Autodesk Fusion 360 part; units mm, degrees
note: some values were not read from the file. Set by a fixed rule: which sketch regions a step uses.
(part 10 of 59)
  spline S52 degree 5 poles (-23.3609, 32.8781) (-23.3596, 32.8757) (-23.3571, 32.871) (-23.3532, 32.8639) (-23.348, 32.8544) (-23.3416, 32.8426) (-23.3351, 32.8308) (-23.3287, 32.819) (-23.3222, 32.8073) (-23.3158, 32.7957) (-23.3094, 32.784) (-23.3029, 32.7724) (-23.2965, 32.7609) (-23.29, 32.7493) (-23.2836, 32.7379) (-23.2771, 32.7264) (-23.2707, 32.715) (-23.2643, 32.7036) (-23.2578, 32.6922) (-23.2514, 32.6809) (-23.245, 32.6697) (-23.2385, 32.6584) (-23.2321, 32.6472) (-23.2257, 32.636) (-23.2193, 32.6249) (-23.2128, 32.6138) (-23.2064, 32.6028) (-23.2, 32.5917) (-23.1936, 32.5808) (-23.1872, 32.5698) (-23.1807, 32.5589) (-23.1743, 32.548) (-23.1679, 32.5372) (-23.1615, 32.5264) (-23.1551, 32.5156) (-23.1487, 32.5049) (-23.1423, 32.4942) (-23.136, 32.4836) (-23.1296, 32.473) (-23.1232, 32.4624) (-23.1168, 32.4518) (-23.1104, 32.4413) (-23.1041, 32.4309) (-23.0977, 32.4205) (-23.0914, 32.4101) (-23.085, 32.3997) (-23.0786, 32.3894) (-23.0723, 32.3791) (-23.066, 32.3689) (-23.0596, 32.3587) (-23.0533, 32.3486) (-23.047, 32.3384) (-23.0406, 32.3284) (-23.0343, 32.3183) (-23.028, 32.3083) (-23.0217, 32.2984) (-23.0154, 32.2884) (-23.0091, 32.2785) (-23.0029, 32.2687) (-22.9966, 32.2589) (-22.9903, 32.2491) (-22.984, 32.2394) (-22.9778, 32.2297) (-22.9715, 32.22) (-22.9653, 32.2104) (-22.9591, 32.2009) (-22.9528, 32.1913) (-22.9466, 32.1818) (-22.9404, 32.1724) (-22.9342, 32.163) (-22.928, 32.1536) (-22.9218, 32.1443) (-22.9156, 32.135) (-22.9095, 32.1257) (-22.9033, 32.1165) (-22.8971, 32.1073) (-22.891, 32.0982) (-22.8849, 32.0891) (-22.8787, 32.0801) (-22.8726, 32.0711) (-22.8665, 32.0621) (-22.8604, 32.0532) (-22.8543, 32.0443) (-22.8483, 32.0354) (-22.8422, 32.0266) (-22.8361, 32.0179) (-22.8301, 32.0091) (-22.8241, 32.0005) (-22.818, 31.9918) (-22.812, 31.9832) (-22.806, 31.9747) (-22.8, 31.9662) (-22.7941, 31.9577) (-22.7881, 31.9493) (-22.7822, 31.9409) (-22.7762, 31.9325) (-22.7703, 31.9242) (-22.7644, 31.916) (-22.7585, 31.9078) (-22.7526, 31.8996) (-22.7467, 31.8914) (-22.7408, 31.8834) (-22.735, 31.8753) (-22.7292, 31.8673) (-22.7233, 31.8593) (-22.7175, 31.8514) (-22.7118, 31.8436) (-22.706, 31.8357) (-22.7002, 31.8279) (-22.6945, 31.8202) (-22.6887, 31.8125) (-22.683, 31.8048) (-22.6773, 31.7972) (-22.6716, 31.7897) (-22.666, 31.7821) (-22.6603, 31.7747) (-22.6547, 31.7672) (-22.6491, 31.7598) (-22.6435, 31.7525) (-22.6379, 31.7452) (-22.6323, 31.7379) (-22.6268, 31.7307) (-22.6212, 31.7236) (-22.6157, 31.7165) (-22.6102, 31.7094) (-22.6048, 31.7024) (-22.5993, 31.6954) (-22.5939, 31.6884) (-22.5884, 31.6815) (-22.583, 31.6747) (-22.5777, 31.6679) (-22.5723, 31.6611) (-22.567, 31.6544) (-22.5617, 31.6478) (-22.5564, 31.6412) (-22.5511, 31.6346) (-22.5458, 31.6281) (-22.5406, 31.6216) (-22.5354, 31.6152) (-22.5302, 31.6088) (-22.525, 31.6025) (-22.5199, 31.5962) (-22.5148, 31.59) (-22.5097, 31.5838) (-22.5046, 31.5776) (-22.4996, 31.5715) (-22.4945, 31.5655) (-22.4895, 31.5595) (-22.4846, 31.5536) (-22.4796, 31.5477) (-22.4747, 31.5418) (-22.4698, 31.536) (-22.4649, 31.5303) (-22.4601, 31.5246) (-22.4553, 31.5189) (-22.4505, 31.5133) (-22.4457, 31.5077) (-22.441, 31.5022) (-22.4363, 31.4968) (-22.4316, 31.4914) (-22.427, 31.486) (-22.4223, 31.4807) (-22.4177, 31.4755) (-22.4132, 31.4703) (-22.4087, 31.4651) (-22.4042, 31.46) (-22.3997, 31.455) (-22.3953, 31.45) (-22.3909, 31.4451) (-22.3865, 31.4402) (-22.3821, 31.4353) (-22.3778, 31.4306) (-22.3736, 31.4258) (-22.3693, 31.4211) (-22.3651, 31.4165) (-22.3609, 31.4119) (-22.3568, 31.4074) (-22.3527, 31.403) (-22.3486, 31.3986) (-22.3446, 31.3942) (-22.3406, 31.3899) (-22.3367, 31.3856) (-22.3328, 31.3814) (-22.3289, 31.3773) (-22.325, 31.3732) (-22.3212, 31.3692) (-22.3175, 31.3652) (-22.3138, 31.3613) (-22.3101, 31.3574) (-22.3065, 31.3536) (-22.3029, 31.3499) (-22.2993, 31.3462) (-22.2958, 31.3426) (-22.2923, 31.339) (-22.2889, 31.3355) (-22.2855, 31.332) (-22.2822, 31.3286) (-22.2789, 31.3252) (-22.2757, 31.322) (-22.2725, 31.3187) (-22.2693, 31.3156) (-22.2662, 31.3124) (-22.2632, 31.3094) (-22.2602, 31.3064) (-22.2572, 31.3035) (-22.2543, 31.3006) (-22.2515, 31.2978) (-22.2487, 31.2951) (-22.2459, 31.2924) (-22.2433, 31.2897) (-22.2406, 31.2872) (-22.238, 31.2847) (-22.2355, 31.2823) (-22.2331, 31.2799) (-22.2307, 31.2776) (-22.2283, 31.2753) (-22.226, 31.2732) (-22.2238, 31.271) (-22.2216, 31.269) (-22.2195, 31.267) (-22.2175, 31.2651) (-22.2155, 31.2632) (-22.2136, 31.2615) (-22.2117, 31.2597) (-22.2099, 31.2581) (-22.2082, 31.2565) (-22.2066, 31.255) (-22.205, 31.2536) (-22.2035, 31.2522) (-22.202, 31.2509) (-22.2007, 31.2497) (-22.1994, 31.2485) (-22.1982, 31.2474) (-22.197, 31.2464) (-22.196, 31.2455) (-22.195, 31.2446) (-22.1941, 31.2438) (-22.1933, 31.2431) (-22.1925, 31.2424) (-22.1919, 31.2419) (-22.1913, 31.2414) (-22.1909, 31.241) (-22.1907, 31.2408) (-22.1905, 31.2407) (-22.1904, 31.2406) knots -1 -1 -1 -1 -1 -1 -0.99583333 -0.99166667 -0.9875 -0.98333333 -0.97916667 -0.975 -0.97083333 -0.96666667 -0.9625 -0.95833333 -0.95416667 -0.95 -0.94583333 -0.94166667 -0.9375 -0.93333333 -0.92916667 -0.925 -0.92083333 -0.91666667 -0.9125 -0.90833333 -0.90416667 -0.9 -0.89583333 -0.89166667 -0.8875 -0.88333333 -0.87916667 -0.875 -0.87083333 -0.86666667 -0.8625 -0.85833333 -0.85416667 -0.85 -0.84583333 -0.84166667 -0.8375 -0.83333333 -0.82916667 -0.825 -0.82083333 -0.81666667 -0.8125 -0.80833333 -0.80416667 -0.8 -0.79583333 -0.79166667 -0.7875 -0.78333333 -0.77916667 -0.775 -0.77083333 -0.76666667 -0.7625 -0.75833333 -0.75416667 -0.75 -0.74583333 -0.74166667 -0.7375 -0.73333333 -0.72916667 -0.725 -0.72083333 -0.71666667 -0.7125 -0.70833333 -0.70416667 -0.7 -0.69583333 -0.69166667 -0.6875 -0.68333333 -0.67916667 -0.675 -0.67083333 -0.66666667 -0.6625 -0.65833333 -0.65416667 -0.65 -0.64583333 -0.64166667 -0.6375 -0.63333333 -0.62916667 -0.625 -0.62083333 -0.61666667 -0.6125 -0.60833333 -0.60416667 -0.6 -0.59583333 -0.59166667 -0.5875 -0.58333333 -0.57916667 -0.575 -0.57083333 -0.56666667 -0.5625 -0.55833333 -0.55416667 -0.55 -0.54583333 -0.54166667 -0.5375 -0.53333333 -0.52916667 -0.525 -0.52083333 -0.51666667 -0.5125 -0.50833333 -0.50416667 -0.5 -0.49583333 -0.49166667 -0.4875 -0.48333333 -0.47916667 -0.475 -0.47083333 -0.46666667 -0.4625 -0.45833333 -0.45416667 -0.45 -0.44583333 -0.44166667 -0.4375 -0.43333333 -0.42916667 -0.425 -0.42083333 -0.41666667 -0.4125 -0.40833333 -0.40416667 -0.4 -0.39583333 -0.39166667 -0.3875 -0.38333333 -0.37916667 -0.375 -0.37083333 -0.36666667 -0.3625 -0.35833333 -0.35416667 -0.35 -0.34583333 -0.34166667 -0.3375 -0.33333333 -0.32916667 -0.325 -0.32083333 -0.31666667 -0.3125 -0.30833333 -0.30416667 -0.3 -0.29583333 -0.29166667 -0.2875 -0.28333333 -0.27916667 -0.275 -0.27083333 -0.26666667 -0.2625 -0.25833333 -0.25416667 -0.25 -0.24583333 -0.24166667 -0.2375 -0.23333333 -0.22916667 -0.225 -0.22083333 -0.21666667 -0.2125 -0.20833333 -0.20416667 -0.2 -0.19583333 -0.19166667 -0.1875 -0.18333333 -0.17916667 -0.175 -0.17083333 -0.16666667 -0.1625 -0.15833333 -0.15416667 -0.15 -0.14583333 -0.14166667 -0.1375 -0.13333333 -0.12916667 -0.125 -0.12083333 -0.11666667 -0.1125 -0.10833333 -0.10416667 -0.1 -0.09583333 -0.09166667 -0.0875 -0.08333333 -0.07916667 -0.075 -0.07083333 -0.06666667 -0.0625 -0.05833333 -0.05416667 -0.05 -0.04583333 -0.04166667 -0.0375 -0.03333333 -0.02916667 -0.025 -0.02083333 -0.01666667 -0.0125 -0.00833333 -0.00416667 0 0 0 0 0 0
  line L120 (-10.8547, 39.1221) -> (-10.9659, 39.3948)
  spline S53 degree 5 poles (-10.0421, 41.8284) (-10.0422, 41.8257) (-10.0423, 41.8203) (-10.0425, 41.8122) (-10.0428, 41.8014) (-10.0431, 41.788) (-10.0434, 41.7745) (-10.0437, 41.7612) (-10.044, 41.7478) (-10.0442, 41.7345) (-10.0445, 41.7212) (-10.0447, 41.7079) (-10.0449, 41.6947) (-10.0451, 41.6815) (-10.0453, 41.6683) (-10.0454, 41.6551) (-10.0455, 41.642) (-10.0457, 41.629) (-10.0458, 41.6159) (-10.0458, 41.6029) (-10.0459, 41.5899) (-10.046, 41.577) (-10.046, 41.5641) (-10.046, 41.5512) (-10.046, 41.5383) (-10.046, 41.5255) (-10.046, 41.5127) (-10.0459, 41.5) (-10.0458, 41.4872) (-10.0458, 41.4745) (-10.0457, 41.4619) (-10.0456, 41.4493) (-10.0454, 41.4367) (-10.0453, 41.4241) (-10.0451, 41.4116) (-10.0449, 41.3991) (-10.0448, 41.3867) (-10.0445, 41.3743) (-10.0443, 41.3619) (-10.0441, 41.3495) (-10.0438, 41.3372) (-10.0436, 41.3249) (-10.0433, 41.3127) (-10.043, 41.3005) (-10.0427, 41.2883) (-10.0423, 41.2762) (-10.042, 41.2641) (-10.0416, 41.252) (-10.0412, 41.24) (-10.0409, 41.228) (-10.0405, 41.216) (-10.04, 41.2041) (-10.0396, 41.1922) (-10.0392, 41.1803) (-10.0387, 41.1685) (-10.0382, 41.1567) (-10.0377, 41.145) (-10.0372, 41.1333) (-10.0367, 41.1216) (-10.0362, 41.11) (-10.0356, 41.0984) (-10.0351, 41.0868) (-10.0345, 41.0753) (-10.0339, 41.0638) (-10.0333, 41.0524) (-10.0327, 41.041) (-10.0321, 41.0296) (-10.0314, 41.0183) (-10.0308, 41.007) (-10.0301, 40.9957) (-10.0294, 40.9845) (-10.0287, 40.9733) (-10.028, 40.9622) (-10.0273, 40.9511) (-10.0266, 40.94) (-10.0258, 40.929) (-10.0251, 40.9181) (-10.0243, 40.9071) (-10.0235, 40.8962) (-10.0227, 40.8854) (-10.0219, 40.8745) (-10.0211, 40.8638) (-10.0203, 40.853) (-10.0195, 40.8423) (-10.0186, 40.8317) (-10.0177, 40.821) (-10.0169, 40.8105) (-10.016, 40.7999) (-10.0151, 40.7894) (-10.0142, 40.779) (-10.0133, 40.7686) (-10.0123, 40.7582) (-10.0114, 40.7479) (-10.0104, 40.7376) (-10.0095, 40.7274) (-10.0085, 40.7172) (-10.0075, 40.707) (-10.0065, 40.6969) (-10.0055, 40.6868) (-10.0045, 40.6768) (-10.0035, 40.6668) (-10.0025, 40.6569) (-10.0014, 40.647) (-10.0004, 40.6372) (-9.9993, 40.6274) (-9.9983, 40.6176) (-9.9972, 40.6079) (-9.9961, 40.5982) (-9.995, 40.5886) (-9.9939, 40.579) (-9.9928, 40.5695) (-9.9916, 40.56) (-9.9905, 40.5506) (-9.9894, 40.5412) (-9.9882, 40.5318) (-9.9871, 40.5225) (-9.9859, 40.5133) (-9.9847, 40.504) (-9.9836, 40.4949) (-9.9824, 40.4858) (-9.9812, 40.4767) (-9.98, 40.4677) (-9.9788, 40.4587) (-9.9776, 40.4498) (-9.9763, 40.4409) (-9.9751, 40.4321) (-9.9739, 40.4233) (-9.9726, 40.4146) (-9.9714, 40.4059) (-9.9701, 40.3973) (-9.9689, 40.3887) (-9.9676, 40.3802) (-9.9664, 40.3717) (-9.9651, 40.3633) (-9.9638, 40.3549) (-9.9625, 40.3466) (-9.9612, 40.3383) (-9.9599, 40.3301) (-9.9586, 40.3219) (-9.9573, 40.3138) (-9.956, 40.3057) (-9.9547, 40.2977) (-9.9534, 40.2898) (-9.9521, 40.2819) (-9.9508, 40.274) (-9.9494, 40.2662) (-9.9481, 40.2585) (-9.9468, 40.2508) (-9.9454, 40.2431) (-9.9441, 40.2356) (-9.9428, 40.228) (-9.9414, 40.2206) (-9.9401, 40.2132) (-9.9387, 40.2058) (-9.9374, 40.1985) (-9.936, 40.1912) (-9.9347, 40.1841) (-9.9333, 40.1769) (-9.932, 40.1698) (-9.9306, 40.1628) (-9.9293, 40.1559) (-9.9279, 40.149) (-9.9266, 40.1421) (-9.9252, 40.1353) (-9.9239, 40.1286) (-9.9225, 40.122) (-9.9212, 40.1154) (-9.9199, 40.1088) (-9.9185, 40.1023) (-9.9172, 40.0959) (-9.9158, 40.0896) (-9.9145, 40.0833) (-9.9132, 40.077) (-9.9118, 40.0709) (-9.9105, 40.0647) (-9.9092, 40.0587) (-9.9079, 40.0527) (-9.9065, 40.0468) (-9.9052, 40.0409) (-9.9039, 40.0352) (-9.9026, 40.0294) (-9.9013, 40.0238) (-9.9, 40.0182) (-9.8987, 40.0127) (-9.8974, 40.0072) (-9.8962, 40.0018) (-9.8949, 39.9965) (-9.8936, 39.9912) (-9.8924, 39.9861) (-9.8911, 39.981) (-9.8899, 39.9759) (-9.8887, 39.9709) (-9.8874, 39.966) (-9.8862, 39.9612) (-9.885, 39.9564) (-9.8838, 39.9517) (-9.8827, 39.9471) (-9.8815, 39.9426) (-9.8803, 39.9381) (-9.8792, 39.9337) (-9.878, 39.9294) (-9.8769, 39.9252) (-9.8758, 39.921) (-9.8747, 39.9169) (-9.8736, 39.9129) (-9.8725, 39.909) (-9.8715, 39.9051) (-9.8704, 39.9013) (-9.8694, 39.8976) (-9.8684, 39.894) (-9.8674, 39.8905) (-9.8664, 39.887) (-9.8654, 39.8837) (-9.8645, 39.8804) (-9.8635, 39.8772) (-9.8626, 39.8741) (-9.8617, 39.871) (-9.8608, 39.8681) (-9.86, 39.8652) (-9.8591, 39.8625) (-9.8583, 39.8598) (-9.8575, 39.8572) (-9.8568, 39.8547) (-9.856, 39.8523) (-9.8553, 39.8499) (-9.8546, 39.8477) (-9.8539, 39.8456) (-9.8533, 39.8435) (-9.8527, 39.8416) (-9.8521, 39.8398) (-9.8515, 39.838) (-9.851, 39.8364) (-9.8505, 39.8348) (-9.85, 39.8334) (-9.8495, 39.832) (-9.8491, 39.8308) (-9.8487, 39.8296) (-9.8484, 39.8286) (-9.8481, 39.8277) (-9.8478, 39.8269) (-9.8475, 39.8262) (-9.8474, 39.8257) (-9.8473, 39.8254) (-9.8472, 39.8252) (-9.8472, 39.8251) knots -1 -1 -1 -1 -1 -1 -0.99583333 -0.99166667 -0.9875 -0.98333333 -0.97916667 -0.975 -0.97083333 -0.96666667 -0.9625 -0.95833333 -0.95416667 -0.95 -0.94583333 -0.94166667 -0.9375 -0.93333333 -0.92916667 -0.925 -0.92083333 -0.91666667 -0.9125 -0.90833333 -0.90416667 -0.9 -0.89583333 -0.89166667 -0.8875 -0.88333333 -0.87916667 -0.875 -0.87083333 -0.86666667 -0.8625 -0.85833333 -0.85416667 -0.85 -0.84583333 -0.84166667 -0.8375 -0.83333333 -0.82916667 -0.825 -0.82083333 -0.81666667 -0.8125 -0.80833333 -0.80416667 -0.8 -0.79583333 -0.79166667 -0.7875 -0.78333333 -0.77916667 -0.775 -0.77083333 -0.76666667 -0.7625 -0.75833333 -0.75416667 -0.75 -0.74583333 -0.74166667 -0.7375 -0.73333333 -0.72916667 -0.725 -0.72083333 -0.71666667 -0.7125 -0.70833333 -0.70416667 -0.7 -0.69583333 -0.69166667 -0.6875 -0.68333333 -0.67916667 -0.675 -0.67083333 -0.66666667 -0.6625 -0.65833333 -0.65416667 -0.65 -0.64583333 -0.64166667 -0.6375 -0.63333333 -0.62916667 -0.625 -0.62083333 -0.61666667 -0.6125 -0.60833333 -0.60416667 -0.6 -0.59583333 -0.59166667 -0.5875 -0.58333333 -0.57916667 -0.575 -0.57083333 -0.56666667 -0.5625 -0.55833333 -0.55416667 -0.55 -0.54583333 -0.54166667 -0.5375 -0.53333333 -0.52916667 -0.525 -0.52083333 -0.51666667 -0.5125 -0.50833333 -0.50416667 -0.5 -0.49583333 -0.49166667 -0.4875 -0.48333333 -0.47916667 -0.475 -0.47083333 -0.46666667 -0.4625 -0.45833333 -0.45416667 -0.45 -0.44583333 -0.44166667 -0.4375 -0.43333333 -0.42916667 -0.425 -0.42083333 -0.41666667 -0.4125 -0.40833333 -0.40416667 -0.4 -0.39583333 -0.39166667 -0.3875 -0.38333333 -0.37916667 -0.375 -0.37083333 -0.36666667 -0.3625 -0.35833333 -0.35416667 -0.35 -0.34583333 -0.34166667 -0.3375 -0.33333333 -0.32916667 -0.325 -0.32083333 -0.31666667 -0.3125 -0.30833333 -0.30416667 -0.3 -0.29583333 -0.29166667 -0.2875 -0.28333333 -0.27916667 -0.275 -0.27083333 -0.26666667 -0.2625 -0.25833333 -0.25416667 -0.25 -0.24583333 -0.24166667 -0.2375 -0.23333333 -0.22916667 -0.225 -0.22083333 -0.21666667 -0.2125 -0.20833333 -0.20416667 -0.2 -0.19583333 -0.19166667 -0.1875 -0.18333333 -0.17916667 -0.175 -0.17083333 -0.16666667 -0.1625 -0.15833333 -0.15416667 -0.15 -0.14583333 -0.14166667 -0.1375 -0.13333333 -0.12916667 -0.125 -0.12083333 -0.11666667 -0.1125 -0.10833333 -0.10416667 -0.1 -0.09583333 -0.09166667 -0.0875 -0.08333333 -0.07916667 -0.075 -0.07083333 -0.06666667 -0.0625 -0.05833333 -0.05416667 -0.05 -0.04583333 -0.04166667 -0.0375 -0.03333333 -0.02916667 -0.025 -0.02083333 -0.01666667 -0.0125 -0.00833333 -0.00416667 0 0 0 0 0 0
  spline S54 degree 5 poles (-22.7084, -8.6029) (-22.7059, -8.6018) (-22.7009, -8.5998) (-22.6934, -8.5967) (-22.6834, -8.5925) (-22.671, -8.5873) (-22.6586, -8.5822) (-22.6462, -8.577) (-22.6339, -8.5718) (-22.6217, -8.5666) (-22.6094, -8.5614) (-22.5972, -8.5562) (-22.585, -8.551) (-22.5729, -8.5458) (-22.5608, -8.5406) (-22.5487, -8.5354) (-22.5367, -8.5302) (-22.5247, -8.525) (-22.5127, -8.5198) (-22.5008, -8.5145) (-22.4889, -8.5093) (-22.4771, -8.5041) (-22.4653, -8.4989) (-22.4535, -8.4937) (-22.4417, -8.4884) (-22.43, -8.4832) (-22.4184, -8.478) (-22.4067, -8.4727) (-22.3951, -8.4675) (-22.3836, -8.4623) (-22.3721, -8.457) (-22.3606, -8.4518) (-22.3491, -8.4466) (-22.3377, -8.4413) (-22.3264, -8.4361) (-22.315, -8.4308) (-22.3037, -8.4256) (-22.2925, -8.4204) (-22.2812, -8.4151) (-22.2701, -8.4099) (-22.2589, -8.4046) (-22.2478, -8.3994) (-22.2367, -8.3942) (-22.2257, -8.3889) (-22.2147, -8.3837) (-22.2038, -8.3784) (-22.1928, -8.3732) (-22.182, -8.368) (-22.1711, -8.3627) (-22.1603, -8.3575) (-22.1496, -8.3523) (-22.1388, -8.347) (-22.1281, -8.3418) (-22.1175, -8.3366) (-22.1069, -8.3313) (-22.0963, -8.3261) (-22.0858, -8.3209) (-22.0753, -8.3157) (-22.0649, -8.3105) (-22.0544, -8.3052) (-22.0441, -8.3) (-22.0337, -8.2948) (-22.0235, -8.2896) (-22.0132, -8.2844) (-22.003, -8.2792) (-21.9928, -8.274) (-21.9827, -8.2688) (-21.9726, -8.2636) (-21.9625, -8.2584) (-21.9525, -8.2532) (-21.9426, -8.248) (-21.9326, -8.2429) (-21.9228, -8.2377) (-21.9129, -8.2325) (-21.9031, -8.2274) (-21.8933, -8.2222) (-21.8836, -8.217) (-21.8739, -8.2119) (-21.8643, -8.2067) (-21.8547, -8.2016) (-21.8451, -8.1965) (-21.8356, -8.1913) (-21.8261, -8.1862) (-21.8167, -8.1811) (-21.8073, -8.176) (-21.798, -8.1709) (-21.7887, -8.1658) (-21.7794, -8.1607) (-21.7702, -8.1556) (-21.761, -8.1505) (-21.7519, -8.1454) (-21.7428, -8.1404) (-21.7337, -8.1353) (-21.7247, -8.1303) (-21.7158, -8.1252) (-21.7068, -8.1202) (-21.698, -8.1152) (-21.6891, -8.1101) (-21.6803, -8.1051) (-21.6716, -8.1001) (-21.6629, -8.0951) (-21.6542, -8.0902) (-21.6456, -8.0852) (-21.6371, -8.0802) (-21.6285, -8.0753) (-21.6201, -8.0703) (-21.6116, -8.0654) (-21.6032, -8.0605) (-21.5949, -8.0555) (-21.5866, -8.0506) (-21.5783, -8.0457) (-21.5701, -8.0409) (-21.5619, -8.036) (-21.5538, -8.0311) (-21.5458, -8.0263) (-21.5377, -8.0214) (-21.5297, -8.0166) (-21.5218, -8.0118) (-21.5139, -8.007) (-21.5061, -8.0022) (-21.4983, -7.9974) (-21.4905, -7.9927) (-21.4828, -7.9879) (-21.4752, -7.9832) (-21.4676, -7.9784) (-21.46, -7.9737) (-21.4525, -7.969) (-21.445, -7.9644) (-21.4376, -7.9597) (-21.4302, -7.955) (-21.4229, -7.9504) (-21.4156, -7.9458) (-21.4084, -7.9412) (-21.4012, -7.9366) (-21.3941, -7.932) (-21.387, -7.9274) (-21.38, -7.9229) (-21.373, -7.9184) (-21.3661, -7.9139) (-21.3592, -7.9094) (-21.3523, -7.9049) (-21.3455, -7.9004) (-21.3388, -7.896) (-21.3321, -7.8916) (-21.3255, -7.8872) (-21.3189, -7.8828) (-21.3124, -7.8784) (-21.3059, -7.8741) (-21.2995, -7.8698) (-21.2931, -7.8655) (-21.2867, -7.8612) (-21.2805, -7.8569) (-21.2742, -7.8527) (-21.2681, -7.8484) (-21.2619, -7.8442) (-21.2559, -7.8401) (-21.2498, -7.8359) (-21.2439, -7.8318) (-21.238, -7.8277) (-21.2321, -7.8236) (-21.2263, -7.8195) (-21.2205, -7.8155) (-21.2148, -7.8115) (-21.2092, -7.8075) (-21.2036, -7.8035) (-21.1981, -7.7996) (-21.1926, -7.7956) (-21.1871, -7.7918) (-21.1818, -7.7879) (-21.1764, -7.7841) (-21.1712, -7.7802) (-21.166, -7.7765) (-21.1608, -7.7727) (-21.1557, -7.769) (-21.1507, -7.7653) (-21.1457, -7.7616) (-21.1408, -7.758) (-21.1359, -7.7544) (-21.1311, -7.7508) (-21.1263, -7.7472) (-21.1216, -7.7437) (-21.117, -7.7402) (-21.1124, -7.7368) (-21.1079, -7.7333) (-21.1034, -7.73) (-21.099, -7.7266) (-21.0947, -7.7233) (-21.0904, -7.72) (-21.0862, -7.7167) (-21.082, -7.7135) (-21.0779, -7.7103) (-21.0739, -7.7072) (-21.0699, -7.7041) (-21.066, -7.701) (-21.0621, -7.698) (-21.0583, -7.695) (-21.0546, -7.692) (-21.0509, -7.6891) (-21.0473, -7.6862) (-21.0437, -7.6834) (-21.0403, -7.6806) (-21.0368, -7.6778) (-21.0335, -7.6751) (-21.0302, -7.6724) (-21.027, -7.6698) (-21.0238, -7.6672) (-21.0207, -7.6647) (-21.0177, -7.6622) (-21.0148, -7.6597) (-21.0119, -7.6573) (-21.009, -7.655) (-21.0063, -7.6527) (-21.0036, -7.6504) (-21.001, -7.6482) (-20.9984, -7.6461) (-20.996, -7.644) (-20.9936, -7.6419) (-20.9912, -7.6399) (-20.989, -7.638) (-20.9868, -7.6361) (-20.9847, -7.6343) (-20.9826, -7.6325) (-20.9806, -7.6308) (-20.9787, -7.6291) (-20.9769, -7.6275) (-20.9752, -7.626) (-20.9735, -7.6245) (-20.9719, -7.623) (-20.9704, -7.6217) (-20.9689, -7.6204) (-20.9675, -7.6192) (-20.9663, -7.618) (-20.9651, -7.6169) (-20.9639, -7.6159) (-20.9629, -7.6149) (-20.9619, -7.614) (-20.961, -7.6132) (-20.9602, -7.6125) (-20.9595, -7.6118) (-20.9589, -7.6112) (-20.9583, -7.6107) (-20.958, -7.6104) (-20.9577, -7.6102) (-20.9576, -7.61) (-20.9575, -7.61) knots -1 -1 -1 -1 -1 -1 -0.99583333 -0.99166667 -0.9875 -0.98333333 -0.97916667 -0.975 -0.97083333 -0.96666667 -0.9625 -0.95833333 -0.95416667 -0.95 -0.94583333 -0.94166667 -0.9375 -0.93333333 -0.92916667 -0.925 -0.92083333 -0.91666667 -0.9125 -0.90833333 -0.90416667 -0.9 -0.89583333 -0.89166667 -0.8875 -0.88333333 -0.87916667 -0.875 -0.87083333 -0.86666667 -0.8625 -0.85833333 -0.85416667 -0.85 -0.84583333 -0.84166667 -0.8375 -0.83333333 -0.82916667 -0.825 -0.82083333 -0.81666667 -0.8125 -0.80833333 -0.80416667 -0.8 -0.79583333 -0.79166667 -0.7875 -0.78333333 -0.77916667 -0.775 -0.77083333 -0.76666667 -0.7625 -0.75833333 -0.75416667 -0.75 -0.74583333 -0.74166667 -0.7375 -0.73333333 -0.72916667 -0.725 -0.72083333 -0.71666667 -0.7125 -0.70833333 -0.70416667 -0.7 -0.69583333 -0.69166667 -0.6875 -0.68333333 -0.67916667 -0.675 -0.67083333 -0.66666667 -0.6625 -0.65833333 -0.65416667 -0.65 -0.64583333 -0.64166667 -0.6375 -0.63333333 -0.62916667 -0.625 -0.62083333 -0.61666667 -0.6125 -0.60833333 -0.60416667 -0.6 -0.59583333 -0.59166667 -0.5875 -0.58333333 -0.57916667 -0.575 -0.57083333 -0.56666667 -0.5625 -0.55833333 -0.55416667 -0.55 -0.54583333 -0.54166667 -0.5375 -0.53333333 -0.52916667 -0.525 -0.52083333 -0.51666667 -0.5125 -0.50833333 -0.50416667 -0.5 -0.49583333 -0.49166667 -0.4875 -0.48333333 -0.47916667 -0.475 -0.47083333 -0.46666667 -0.4625 -0.45833333 -0.45416667 -0.45 -0.44583333 -0.44166667 -0.4375 -0.43333333 -0.42916667 -0.425 -0.42083333 -0.41666667 -0.4125 -0.40833333 -0.40416667 -0.4 -0.39583333 -0.39166667 -0.3875 -0.38333333 -0.37916667 -0.375 -0.37083333 -0.36666667 -0.3625 -0.35833333 -0.35416667 -0.35 -0.34583333 -0.34166667 -0.3375 -0.33333333 -0.32916667 -0.325 -0.32083333 -0.31666667 -0.3125 -0.30833333 -0.30416667 -0.3 -0.29583333 -0.29166667 -0.2875 -0.28333333 -0.27916667 -0.275 -0.27083333 -0.26666667 -0.2625 -0.25833333 -0.25416667 -0.25 -0.24583333 -0.24166667 -0.2375 -0.23333333 -0.22916667 -0.225 -0.22083333 -0.21666667 -0.2125 -0.20833333 -0.20416667 -0.2 -0.19583333 -0.19166667 -0.1875 -0.18333333 -0.17916667 -0.175 -0.17083333 -0.16666667 -0.1625 -0.15833333 -0.15416667 -0.15 -0.14583333 -0.14166667 -0.1375 -0.13333333 -0.12916667 -0.125 -0.12083333 -0.11666667 -0.1125 -0.10833333 -0.10416667 -0.1 -0.09583333 -0.09166667 -0.0875 -0.08333333 -0.07916667 -0.075 -0.07083333 -0.06666667 -0.0625 -0.05833333 -0.05416667 -0.05 -0.04583333 -0.04166667 -0.0375 -0.03333333 -0.02916667 -0.025 -0.02083333 -0.01666667 -0.0125 -0.00833333 -0.00416667 0 0 0 0 0 0
  spline S55 degree 5 poles (-8.0948, 40.3945) (-8.0948, 40.3946) (-8.0948, 40.3948) (-8.0949, 40.3951) (-8.0951, 40.3956) (-8.0953, 40.3963) (-8.0956, 40.3971) (-8.0958, 40.398) (-8.0962, 40.3991) (-8.0965, 40.4002) (-8.0969, 40.4015) (-8.0973, 40.4028) (-8.0978, 40.4043) (-8.0983, 40.4058) (-8.0988, 40.4075) (-8.0994, 40.4092) (-8.1, 40.4111) (-8.1007, 40.413) (-8.1013, 40.415) (-8.102, 40.4172) (-8.1028, 40.4194) (-8.1036, 40.4217) (-8.1044, 40.4241) (-8.1052, 40.4265) (-8.1061, 40.4291) (-8.107, 40.4318) (-8.108, 40.4345) (-8.109, 40.4373) (-8.11, 40.4402) (-8.1111, 40.4432) (-8.1121, 40.4462) (-8.1133, 40.4494) (-8.1144, 40.4526) (-8.1156, 40.4559) (-8.1169, 40.4593) (-8.1181, 40.4627) (-8.1194, 40.4662) (-8.1208, 40.4698) (-8.1222, 40.4735) (-8.1236, 40.4772) (-8.125, 40.4811) (-8.1265, 40.4849) (-8.128, 40.4889) (-8.1295, 40.4929) (-8.1311, 40.497) (-8.1327, 40.5012) (-8.1344, 40.5054) (-8.1361, 40.5097) (-8.1378, 40.5141) (-8.1395, 40.5185) (-8.1413, 40.523) (-8.1432, 40.5276) (-8.145, 40.5322) (-8.1469, 40.5369) (-8.1488, 40.5416) (-8.1508, 40.5464) (-8.1528, 40.5513) (-8.1548, 40.5562) (-8.1569, 40.5612) (-8.159, 40.5663) (-8.1611, 40.5714) (-8.1633, 40.5765) (-8.1655, 40.5818) (-8.1677, 40.587) (-8.17, 40.5924) (-8.1723, 40.5978) (-8.1747, 40.6032) (-8.177, 40.6087) (-8.1795, 40.6143) (-8.1819, 40.6199) (-8.1844, 40.6256) (-8.1869, 40.6313) (-8.1895, 40.6371) (-8.192, 40.6429) (-8.1947, 40.6488) (-8.1973, 40.6547) (-8.2, 40.6607) (-8.2027, 40.6667) (-8.2055, 40.6728) (-8.2083, 40.679) (-8.2111, 40.6851) (-8.214, 40.6914) (-8.2169, 40.6977) (-8.2198, 40.704) (-8.2227, 40.7104) (-8.2257, 40.7168) (-8.2288, 40.7233) (-8.2318, 40.7298) (-8.2349, 40.7363) (-8.2381, 40.7429) (-8.2412, 40.7496) (-8.2445, 40.7563) (-8.2477, 40.763) (-8.251, 40.7698) (-8.2543, 40.7767) (-8.2576, 40.7835) (-8.261, 40.7905) (-8.2644, 40.7974) (-8.2678, 40.8044) (-8.2713, 40.8115) (-8.2748, 40.8186) (-8.2784, 40.8257) (-8.282, 40.8329) (-8.2856, 40.8401) (-8.2892, 40.8473) (-8.2929, 40.8546) (-8.2966, 40.8619) (-8.3004, 40.8693) (-8.3042, 40.8767) (-8.308, 40.8842) (-8.3118, 40.8917) (-8.3157, 40.8992) (-8.3196, 40.9068) (-8.3236, 40.9144) (-8.3276, 40.922) (-8.3316, 40.9297) (-8.3357, 40.9374) (-8.3398, 40.9452) (-8.3439, 40.9529) (-8.348, 40.9608) (-8.3522, 40.9686) (-8.3565, 40.9765) (-8.3607, 40.9845) (-8.365, 40.9924) (-8.3693, 41.0004) (-8.3737, 41.0085) (-8.3781, 41.0165) (-8.3825, 41.0246) (-8.387, 41.0328) (-8.3915, 41.0409) (-8.396, 41.0491) (-8.4006, 41.0574) (-8.4052, 41.0657) (-8.4098, 41.074) (-8.4145, 41.0823) (-8.4192, 41.0907) (-8.4239, 41.0991) (-8.4287, 41.1075) (-8.4335, 41.116) (-8.4384, 41.1244) (-8.4432, 41.133) (-8.4481, 41.1415) (-8.4531, 41.1501) (-8.458, 41.1587) (-8.463, 41.1674) (-8.4681, 41.176) (-8.4732, 41.1847) (-8.4783, 41.1935) (-8.4834, 41.2022) (-8.4886, 41.211) (-8.4938, 41.2199) (-8.499, 41.2287) (-8.5043, 41.2376) (-8.5096, 41.2465) (-8.515, 41.2554) (-8.5203, 41.2644) (-8.5257, 41.2734) (-8.5312, 41.2824) (-8.5367, 41.2914) (-8.5422, 41.3005) (-8.5477, 41.3096) (-8.5533, 41.3187) (-8.5589, 41.3279) (-8.5645, 41.337) (-8.5702, 41.3462) (-8.5759, 41.3555) (-8.5817, 41.3647) (-8.5874, 41.374) (-8.5932, 41.3833) (-8.5991, 41.3926) (-8.605, 41.402) (-8.6109, 41.4113) (-8.6168, 41.4207) (-8.6228, 41.4302) (-8.6288, 41.4396) (-8.6348, 41.4491) (-8.6409, 41.4586) (-8.647, 41.4681) (-8.6532, 41.4776) (-8.6593, 41.4872) (-8.6656, 41.4968) (-8.6718, 41.5064) (-8.6781, 41.516) (-8.6844, 41.5257) (-8.6907, 41.5354) (-8.6971, 41.5451) (-8.7035, 41.5548) (-8.7099, 41.5646) (-8.7164, 41.5743) (-8.7229, 41.5841) (-8.7295, 41.5939) (-8.736, 41.6037) (-8.7426, 41.6136) (-8.7493, 41.6235) (-8.7559, 41.6334) (-8.7626, 41.6433) (-8.7694, 41.6532) (-8.7762, 41.6632) (-8.783, 41.6731) (-8.7898, 41.6831) (-8.7967, 41.6932) (-8.8036, 41.7032) (-8.8105, 41.7132) (-8.8175, 41.7233) (-8.8245, 41.7334) (-8.8315, 41.7435) (-8.8386, 41.7537) (-8.8457, 41.7638) (-8.8528, 41.774) (-8.86, 41.7842) (-8.8671, 41.7944) (-8.8744, 41.8046) (-8.8816, 41.8148) (-8.8889, 41.8251) (-8.8963, 41.8354) (-8.9036, 41.8457) (-8.911, 41.856) (-8.9184, 41.8663) (-8.9259, 41.8766) (-8.9334, 41.887) (-8.9409, 41.8974) (-8.9485, 41.9078) (-8.956, 41.9182) (-8.9637, 41.9286) (-8.9713, 41.9391) (-8.979, 41.9495) (-8.9867, 41.96) (-8.9945, 41.9705) (-9.0022, 41.981) (-9.0101, 41.9915) (-9.0179, 42.0021) (-9.0258, 42.0127) (-9.0337, 42.0232) (-9.0416, 42.0338) (-9.0496, 42.0444) (-9.0576, 42.055) (-9.0657, 42.0657) (-9.0737, 42.0763) (-9.0818, 42.087) (-9.09, 42.0977) (-9.0981, 42.1084) (-9.1047, 42.1169) (-9.1096, 42.1234) (-9.1129, 42.1276) (-9.1146, 42.1298) knots 0 0 0 0 0 0 0.00416667 0.00833333 0.0125 0.01666667 0.02083333 0.025 0.02916667 0.03333333 0.0375 0.04166667 0.04583333 0.05 0.05416667 0.05833333 0.0625 0.06666667 0.07083333 0.075 0.07916667 0.08333333 0.0875 0.09166667 0.09583333 0.1 0.10416667 0.10833333 0.1125 0.11666667 0.12083333 0.125 0.12916667 0.13333333 0.1375 0.14166667 0.14583333 0.15 0.15416667 0.15833333 0.1625 0.16666667 0.17083333 0.175 0.17916667 0.18333333 0.1875 0.19166667 0.19583333 0.2 0.20416667 0.20833333 0.2125 0.21666667 0.22083333 0.225 0.22916667 0.23333333 0.2375 0.24166667 0.24583333 0.25 0.25416667 0.25833333 0.2625 0.26666667 0.27083333 0.275 0.27916667 0.28333333 0.2875 0.29166667 0.29583333 0.3 0.30416667 0.30833333 0.3125 0.31666667 0.32083333 0.325 0.32916667 0.33333333 0.3375 0.34166667 0.34583333 0.35 0.35416667 0.35833333 0.3625 0.36666667 0.37083333 0.375 0.37916667 0.38333333 0.3875 0.39166667 0.39583333 0.4 0.40416667 0.40833333 0.4125 0.41666667 0.42083333 0.425 0.42916667 0.43333333 0.4375 0.44166667 0.44583333 0.45 0.45416667 0.45833333 0.4625 0.46666667 0.47083333 0.475 0.47916667 0.48333333 0.4875 0.49166667 0.49583333 0.5 0.50416667 0.50833333 0.5125 0.51666667 0.52083333 0.525 0.52916667 0.53333333 0.5375 0.54166667 0.54583333 0.55 0.55416667 0.55833333 0.5625 0.56666667 0.57083333 0.575 0.57916667 0.58333333 0.5875 0.59166667 0.59583333 0.6 0.60416667 0.60833333 0.6125 0.61666667 0.62083333 0.625 0.62916667 0.63333333 0.6375 0.64166667 0.64583333 0.65 0.65416667 0.65833333 0.6625 0.66666667 0.67083333 0.675 0.67916667 0.68333333 0.6875 0.69166667 0.69583333 0.7 0.70416667 0.70833333 0.7125 0.71666667 0.72083333 0.725 0.72916667 0.73333333 0.7375 0.74166667 0.74583333 0.75 0.75416667 0.75833333 0.7625 0.76666667 0.77083333 0.775 0.77916667 0.78333333 0.7875 0.79166667 0.79583333 0.8 0.80416667 0.80833333 0.8125 0.81666667 0.82083333 0.825 0.82916667 0.83333333 0.8375 0.84166667 0.84583333 0.85 0.85416667 0.85833333 0.8625 0.86666667 0.87083333 0.875 0.87916667 0.88333333 0.8875 0.89166667 0.89583333 0.9 0.90416667 0.90833333 0.9125 0.91666667 0.92083333 0.925 0.92916667 0.93333333 0.9375 0.94166667 0.94583333 0.95 0.95416667 0.95833333 0.9625 0.96666667 0.97083333 0.975 0.97916667 0.98333333 0.9875 0.99166667 0.99583333 1 1 1 1 1 1
  spline S56 degree 5 poles (-5.1346, 41.0878) (-5.1347, 41.0879) (-5.1347, 41.0881) (-5.1348, 41.0884) (-5.1349, 41.0889) (-5.135, 41.0896) (-5.1352, 41.0905) (-5.1354, 41.0915) (-5.1356, 41.0925) (-5.1358, 41.0937) (-5.1361, 41.095) (-5.1363, 41.0964) (-5.1367, 41.0979) (-5.137, 41.0995) (-5.1374, 41.1012) (-5.1377, 41.103) (-5.1381, 41.1049) (-5.1386, 41.1069) (-5.139, 41.1089) (-5.1395, 41.1111) (-5.14, 41.1134) (-5.1406, 41.1158) (-5.1411, 41.1182) (-5.1417, 41.1208) (-5.1423, 41.1234) (-5.143, 41.1262) (-5.1436, 41.129) (-5.1443, 41.1319) (-5.145, 41.1349) (-5.1458, 41.1379) (-5.1465, 41.1411) (-5.1473, 41.1443) (-5.1481, 41.1477) (-5.149, 41.1511) (-5.1499, 41.1545) (-5.1508, 41.1581) (-5.1517, 41.1617) (-5.1527, 41.1655) (-5.1536, 41.1693) (-5.1546, 41.1731) (-5.1557, 41.1771) (-5.1567, 41.1811) (-5.1578, 41.1852) (-5.1589, 41.1893) (-5.1601, 41.1936) (-5.1613, 41.1979) (-5.1625, 41.2023) (-5.1637, 41.2067) (-5.1649, 41.2112) (-5.1662, 41.2158) (-5.1675, 41.2205) (-5.1689, 41.2252) (-5.1702, 41.23) (-5.1716, 41.2349) (-5.173, 41.2398) (-5.1745, 41.2448) (-5.176, 41.2498) (-5.1775, 41.2549) (-5.179, 41.2601) (-5.1806, 41.2654) (-5.1822, 41.2707) (-5.1838, 41.276) (-5.1854, 41.2815) (-5.1871, 41.2869) (-5.1888, 41.2925) (-5.1905, 41.2981) (-5.1923, 41.3038) (-5.1941, 41.3095) (-5.1959, 41.3153) (-5.1978, 41.3211) (-5.1996, 41.327) (-5.2015, 41.333) (-5.2035, 41.339) (-5.2054, 41.3451) (-5.2074, 41.3512) (-5.2094, 41.3573) (-5.2115, 41.3636) (-5.2136, 41.3699) (-5.2157, 41.3762) (-5.2178, 41.3826) (-5.22, 41.389) (-5.2222, 41.3955) (-5.2244, 41.4021) (-5.2266, 41.4087) (-5.2289, 41.4153) (-5.2312, 41.422) (-5.2336, 41.4288) (-5.2359, 41.4356) (-5.2383, 41.4424) (-5.2408, 41.4493) (-5.2432, 41.4563) (-5.2457, 41.4633) (-5.2482, 41.4703) (-5.2508, 41.4774) (-5.2533, 41.4846) (-5.2559, 41.4918) (-5.2586, 41.499) (-5.2612, 41.5063) (-5.2639, 41.5136) (-5.2666, 41.521) (-5.2694, 41.5284) (-5.2722, 41.5358) (-5.275, 41.5433) (-5.2778, 41.5509) (-5.2807, 41.5585) (-5.2836, 41.5661) (-5.2865, 41.5738) (-5.2895, 41.5815) (-5.2925, 41.5893) (-5.2955, 41.5971) (-5.2986, 41.605) (-5.3016, 41.6129) (-5.3047, 41.6208) (-5.3079, 41.6288) (-5.3111, 41.6368) (-5.3143, 41.6448) (-5.3175, 41.6529) (-5.3207, 41.6611) (-5.324, 41.6692) (-5.3273, 41.6775) (-5.3307, 41.6857) (-5.3341, 41.694) (-5.3375, 41.7023) (-5.3409, 41.7107) (-5.3444, 41.7191) (-5.3479, 41.7276) (-5.3514, 41.7361) (-5.355, 41.7446) (-5.3586, 41.7531) (-5.3622, 41.7617) (-5.3658, 41.7704) (-5.3695, 41.779) (-5.3732, 41.7878) (-5.377, 41.7965) (-5.3807, 41.8053) (-5.3846, 41.8141) (-5.3884, 41.8229) (-5.3922, 41.8318) (-5.3961, 41.8407) (-5.4001, 41.8497) (-5.404, 41.8587) (-5.408, 41.8677) (-5.412, 41.8767) (-5.4161, 41.8858) (-5.4201, 41.895) (-5.4242, 41.9041) (-5.4284, 41.9133) (-5.4325, 41.9225) (-5.4367, 41.9318) (-5.441, 41.941) (-5.4452, 41.9504) (-5.4495, 41.9597) (-5.4538, 41.9691) (-5.4582, 41.9785) (-5.4625, 41.9879) (-5.467, 41.9974) (-5.4714, 42.0069) (-5.4759, 42.0165) (-5.4804, 42.026) (-5.4849, 42.0356) (-5.4895, 42.0452) (-5.494, 42.0549) (-5.4987, 42.0646) (-5.5033, 42.0743) (-5.508, 42.084) (-5.5127, 42.0938) (-5.5175, 42.1036) (-5.5222, 42.1134) (-5.527, 42.1233) (-5.5319, 42.1332) (-5.5367, 42.1431) (-5.5416, 42.153) (-5.5466, 42.163) (-5.5515, 42.173) (-5.5565, 42.183) (-5.5615, 42.1931) (-5.5666, 42.2032) (-5.5717, 42.2133) (-5.5768, 42.2234) (-5.5819, 42.2336) (-5.5871, 42.2437) (-5.5923, 42.254) (-5.5975, 42.2642) (-5.6028, 42.2745) (-5.6081, 42.2847) (-5.6134, 42.2951) (-5.6188, 42.3054) (-5.6242, 42.3158) (-5.6296, 42.3262) (-5.635, 42.3366) (-5.6405, 42.347) (-5.646, 42.3575) (-5.6515, 42.368) (-5.6571, 42.3785) (-5.6627, 42.389) (-5.6683, 42.3996) (-5.674, 42.4102) (-5.6797, 42.4208) (-5.6854, 42.4314) (-5.6912, 42.4421) (-5.697, 42.4527) (-5.7028, 42.4634) (-5.7086, 42.4742) (-5.7145, 42.4849) (-5.7204, 42.4957) (-5.7263, 42.5065) (-5.7323, 42.5173) (-5.7383, 42.5281) (-5.7443, 42.539) (-5.7504, 42.5499) (-5.7565, 42.5608) (-5.7626, 42.5717) (-5.7688, 42.5826) (-5.7749, 42.5936) (-5.7811, 42.6046) (-5.7874, 42.6156) (-5.7937, 42.6266) (-5.8, 42.6377) (-5.8063, 42.6487) (-5.8127, 42.6598) (-5.8191, 42.6709) (-5.8255, 42.6821) (-5.8319, 42.6932) (-5.8384, 42.7044) (-5.8449, 42.7156) (-5.8515, 42.7268) (-5.8581, 42.738) (-5.8647, 42.7492) (-5.8713, 42.7605) (-5.878, 42.7718) (-5.8847, 42.7831) (-5.8914, 42.7944) (-5.8982, 42.8058) (-5.905, 42.8171) (-5.9118, 42.8285) (-5.9187, 42.8399) (-5.9255, 42.8513) (-5.9325, 42.8628) (-5.9394, 42.8742) (-5.9464, 42.8857) (-5.9534, 42.8972) (-5.959, 42.9064) (-5.9633, 42.9133) (-5.9661, 42.9179) (-5.9675, 42.9202) knots 0 0 0 0 0 0 0.00416667 0.00833333 0.0125 0.01666667 0.02083333 0.025 0.02916667 0.03333333 0.0375 0.04166667 0.04583333 0.05 0.05416667 0.05833333 0.0625 0.06666667 0.07083333 0.075 0.07916667 0.08333333 0.0875 0.09166667 0.09583333 0.1 0.10416667 0.10833333 0.1125 0.11666667 0.12083333 0.125 0.12916667 0.13333333 0.1375 0.14166667 0.14583333 0.15 0.15416667 0.15833333 0.1625 0.16666667 0.17083333 0.175 0.17916667 0.18333333 0.1875 0.19166667 0.19583333 0.2 0.20416667 0.20833333 0.2125 0.21666667 0.22083333 0.225 0.22916667 0.23333333 0.2375 0.24166667 0.24583333 0.25 0.25416667 0.25833333 0.2625 0.26666667 0.27083333 0.275 0.27916667 0.28333333 0.2875 0.29166667 0.29583333 0.3 0.30416667 0.30833333 0.3125 0.31666667 0.32083333 0.325 0.32916667 0.33333333 0.3375 0.34166667 0.34583333 0.35 0.35416667 0.35833333 0.3625 0.36666667 0.37083333 0.375 0.37916667 0.38333333 0.3875 0.39166667 0.39583333 0.4 0.40416667 0.40833333 0.4125 0.41666667 0.42083333 0.425 0.42916667 0.43333333 0.4375 0.44166667 0.44583333 0.45 0.45416667 0.45833333 0.4625 0.46666667 0.47083333 0.475 0.47916667 0.48333333 0.4875 0.49166667 0.49583333 0.5 0.50416667 0.50833333 0.5125 0.51666667 0.52083333 0.525 0.52916667 0.53333333 0.5375 0.54166667 0.54583333 0.55 0.55416667 0.55833333 0.5625 0.56666667 0.57083333 0.575 0.57916667 0.58333333 0.5875 0.59166667 0.59583333 0.6 0.60416667 0.60833333 0.6125 0.61666667 0.62083333 0.625 0.62916667 0.63333333 0.6375 0.64166667 0.64583333 0.65 0.65416667 0.65833333 0.6625 0.66666667 0.67083333 0.675 0.67916667 0.68333333 0.6875 0.69166667 0.69583333 0.7 0.70416667 0.70833333 0.7125 0.71666667 0.72083333 0.725 0.72916667 0.73333333 0.7375 0.74166667 0.74583333 0.75 0.75416667 0.75833333 0.7625 0.76666667 0.77083333 0.775 0.77916667 0.78333333 0.7875 0.79166667 0.79583333 0.8 0.80416667 0.80833333 0.8125 0.81666667 0.82083333 0.825 0.82916667 0.83333333 0.8375 0.84166667 0.84583333 0.85 0.85416667 0.85833333 0.8625 0.86666667 0.87083333 0.875 0.87916667 0.88333333 0.8875 0.89166667 0.89583333 0.9 0.90416667 0.90833333 0.9125 0.91666667 0.92083333 0.925 0.92916667 0.93333333 0.9375 0.94166667 0.94583333 0.95 0.95416667 0.95833333 0.9625 0.96666667 0.97083333 0.975 0.97916667 0.98333333 0.9875 0.99166667 0.99583333 1 1 1 1 1 1
  spline S57 degree 5 poles (-22.1904, -6.2406) (-22.1905, -6.2407) (-22.1907, -6.2408) (-22.1909, -6.241) (-22.1913, -6.2414) (-22.1919, -6.2419) (-22.1925, -6.2424) (-22.1933, -6.2431) (-22.1941, -6.2438) (-22.195, -6.2446) (-22.196, -6.2455) (-22.197, -6.2464) (-22.1982, -6.2474) (-22.1994, -6.2485) (-22.2007, -6.2497) (-22.202, -6.2509) (-22.2035, -6.2522) (-22.205, -6.2536) (-22.2066, -6.255) (-22.2082, -6.2565) (-22.2099, -6.2581) (-22.2117, -6.2597) (-22.2136, -6.2615) (-22.2155, -6.2632) (-22.2175, -6.2651) (-22.2195, -6.267) (-22.2216, -6.269) (-22.2238, -6.271) (-22.226, -6.2732) (-22.2283, -6.2753) (-22.2307, -6.2776) (-22.2331, -6.2799) (-22.2355, -6.2823) (-22.238, -6.2847) (-22.2406, -6.2872) (-22.2433, -6.2897) (-22.2459, -6.2924) (-22.2487, -6.2951) (-22.2515, -6.2978) (-22.2543, -6.3006) (-22.2572, -6.3035) (-22.2602, -6.3064) (-22.2632, -6.3094) (-22.2662, -6.3124) (-22.2693, -6.3156) (-22.2725, -6.3187) (-22.2757, -6.322) (-22.2789, -6.3252) (-22.2822, -6.3286) (-22.2855, -6.332) (-22.2889, -6.3355) (-22.2923, -6.339) (-22.2958, -6.3426) (-22.2993, -6.3462) (-22.3029, -6.3499) (-22.3065, -6.3536) (-22.3101, -6.3574) (-22.3138, -6.3613) (-22.3175, -6.3652) (-22.3212, -6.3692) (-22.325, -6.3732) (-22.3289, -6.3773) (-22.3328, -6.3814) (-22.3367, -6.3856) (-22.3406, -6.3899) (-22.3446, -6.3942) (-22.3486, -6.3986) (-22.3527, -6.403) (-22.3568, -6.4074) (-22.3609, -6.4119) (-22.3651, -6.4165) (-22.3693, -6.4211) (-22.3736, -6.4258) (-22.3778, -6.4306) (-22.3821, -6.4353) (-22.3865, -6.4402) (-22.3909, -6.4451) (-22.3953, -6.45) (-22.3997, -6.455) (-22.4042, -6.46) (-22.4087, -6.4651) (-22.4132, -6.4703) (-22.4177, -6.4755) (-22.4223, -6.4807) (-22.427, -6.486) (-22.4316, -6.4914) (-22.4363, -6.4968) (-22.441, -6.5022) (-22.4457, -6.5077) (-22.4505, -6.5133) (-22.4553, -6.5189) (-22.4601, -6.5246) (-22.4649, -6.5303) (-22.4698, -6.536) (-22.4747, -6.5418) (-22.4796, -6.5477) (-22.4846, -6.5536) (-22.4895, -6.5595) (-22.4945, -6.5655) (-22.4996, -6.5715) (-22.5046, -6.5776) (-22.5097, -6.5838) (-22.5148, -6.59) (-22.5199, -6.5962) (-22.525, -6.6025) (-22.5302, -6.6088) (-22.5354, -6.6152) (-22.5406, -6.6216) (-22.5458, -6.6281) (-22.5511, -6.6346) (-22.5564, -6.6412) (-22.5617, -6.6478) (-22.567, -6.6544) (-22.5723, -6.6611) (-22.5777, -6.6679) (-22.583, -6.6747) (-22.5884, -6.6815) (-22.5939, -6.6884) (-22.5993, -6.6954) (-22.6048, -6.7024) (-22.6102, -6.7094) (-22.6157, -6.7165) (-22.6212, -6.7236) (-22.6268, -6.7307) (-22.6323, -6.7379) (-22.6379, -6.7452) (-22.6435, -6.7525) (-22.6491, -6.7598) (-22.6547, -6.7672) (-22.6603, -6.7747) (-22.666, -6.7821) (-22.6716, -6.7897) (-22.6773, -6.7972) (-22.683, -6.8048) (-22.6887, -6.8125) (-22.6945, -6.8202) (-22.7002, -6.8279) (-22.706, -6.8357) (-22.7118, -6.8436) (-22.7175, -6.8514) (-22.7233, -6.8593) (-22.7292, -6.8673) (-22.735, -6.8753) (-22.7408, -6.8834) (-22.7467, -6.8914) (-22.7526, -6.8996) (-22.7585, -6.9078) (-22.7644, -6.916) (-22.7703, -6.9242) (-22.7762, -6.9325) (-22.7822, -6.9409) (-22.7881, -6.9493) (-22.7941, -6.9577) (-22.8, -6.9662) (-22.806, -6.9747) (-22.812, -6.9832) (-22.818, -6.9918) (-22.8241, -7.0005) (-22.8301, -7.0091) (-22.8361, -7.0179) (-22.8422, -7.0266) (-22.8483, -7.0354) (-22.8543, -7.0443) (-22.8604, -7.0532) (-22.8665, -7.0621) (-22.8726, -7.0711) (-22.8787, -7.0801) (-22.8849, -7.0891) (-22.891, -7.0982) (-22.8971, -7.1073) (-22.9033, -7.1165) (-22.9095, -7.1257) (-22.9156, -7.135) (-22.9218, -7.1443) (-22.928, -7.1536) (-22.9342, -7.163) (-22.9404, -7.1724) (-22.9466, -7.1818) (-22.9528, -7.1913) (-22.9591, -7.2009) (-22.9653, -7.2104) (-22.9715, -7.22) (-22.9778, -7.2297) (-22.984, -7.2394) (-22.9903, -7.2491) (-22.9966, -7.2589) (-23.0029, -7.2687) (-23.0091, -7.2785) (-23.0154, -7.2884) (-23.0217, -7.2984) (-23.028, -7.3083) (-23.0343, -7.3183) (-23.0406, -7.3284) (-23.047, -7.3384) (-23.0533, -7.3486) (-23.0596, -7.3587) (-23.066, -7.3689) (-23.0723, -7.3791) (-23.0786, -7.3894) (-23.085, -7.3997) (-23.0914, -7.4101) (-23.0977, -7.4205) (-23.1041, -7.4309) (-23.1104, -7.4413) (-23.1168, -7.4518) (-23.1232, -7.4624) (-23.1296, -7.473) (-23.136, -7.4836) (-23.1423, -7.4942) (-23.1487, -7.5049) (-23.1551, -7.5156) (-23.1615, -7.5264) (-23.1679, -7.5372) (-23.1743, -7.548) (-23.1807, -7.5589) (-23.1872, -7.5698) (-23.1936, -7.5808) (-23.2, -7.5917) (-23.2064, -7.6028) (-23.2128, -7.6138) (-23.2193, -7.6249) (-23.2257, -7.636) (-23.2321, -7.6472) (-23.2385, -7.6584) (-23.245, -7.6697) (-23.2514, -7.6809) (-23.2578, -7.6922) (-23.2643, -7.7036) (-23.2707, -7.715) (-23.2771, -7.7264) (-23.2836, -7.7379) (-23.29, -7.7493) (-23.2965, -7.7609) (-23.3029, -7.7724) (-23.3094, -7.784) (-23.3158, -7.7957) (-23.3222, -7.8073) (-23.3287, -7.819) (-23.3351, -7.8308) (-23.3416, -7.8426) (-23.348, -7.8544) (-23.3532, -7.8639) (-23.3571, -7.871) (-23.3596, -7.8757) (-23.3609, -7.8781) knots 0 0 0 0 0 0 0.00416667 0.00833333 0.0125 0.01666667 0.02083333 0.025 0.02916667 0.03333333 0.0375 0.04166667 0.04583333 0.05 0.05416667 0.05833333 0.0625 0.06666667 0.07083333 0.075 0.07916667 0.08333333 0.0875 0.09166667 0.09583333 0.1 0.10416667 0.10833333 0.1125 0.11666667 0.12083333 0.125 0.12916667 0.13333333 0.1375 0.14166667 0.14583333 0.15 0.15416667 0.15833333 0.1625 0.16666667 0.17083333 0.175 0.17916667 0.18333333 0.1875 0.19166667 0.19583333 0.2 0.20416667 0.20833333 0.2125 0.21666667 0.22083333 0.225 0.22916667 0.23333333 0.2375 0.24166667 0.24583333 0.25 0.25416667 0.25833333 0.2625 0.26666667 0.27083333 0.275 0.27916667 0.28333333 0.2875 0.29166667 0.29583333 0.3 0.30416667 0.30833333 0.3125 0.31666667 0.32083333 0.325 0.32916667 0.33333333 0.3375 0.34166667 0.34583333 0.35 0.35416667 0.35833333 0.3625 0.36666667 0.37083333 0.375 0.37916667 0.38333333 0.3875 0.39166667 0.39583333 0.4 0.40416667 0.40833333 0.4125 0.41666667 0.42083333 0.425 0.42916667 0.43333333 0.4375 0.44166667 0.44583333 0.45 0.45416667 0.45833333 0.4625 0.46666667 0.47083333 0.475 0.47916667 0.48333333 0.4875 0.49166667 0.49583333 0.5 0.50416667 0.50833333 0.5125 0.51666667 0.52083333 0.525 0.52916667 0.53333333 0.5375 0.54166667 0.54583333 0.55 0.55416667 0.55833333 0.5625 0.56666667 0.57083333 0.575 0.57916667 0.58333333 0.5875 0.59166667 0.59583333 0.6 0.60416667 0.60833333 0.6125 0.61666667 0.62083333 0.625 0.62916667 0.63333333 0.6375 0.64166667 0.64583333 0.65 0.65416667 0.65833333 0.6625 0.66666667 0.67083333 0.675 0.67916667 0.68333333 0.6875 0.69166667 0.69583333 0.7 0.70416667 0.70833333 0.7125 0.71666667 0.72083333 0.725 0.72916667 0.73333333 0.7375 0.74166667 0.74583333 0.75 0.75416667 0.75833333 0.7625 0.76666667 0.77083333 0.775 0.77916667 0.78333333 0.7875 0.79166667 0.79583333 0.8 0.80416667 0.80833333 0.8125 0.81666667 0.82083333 0.825 0.82916667 0.83333333 0.8375 0.84166667 0.84583333 0.85 0.85416667 0.85833333 0.8625 0.86666667 0.87083333 0.875 0.87916667 0.88333333 0.8875 0.89166667 0.89583333 0.9 0.90416667 0.90833333 0.9125 0.91666667 0.92083333 0.925 0.92916667 0.93333333 0.9375 0.94166667 0.94583333 0.95 0.95416667 0.95833333 0.9625 0.96666667 0.97083333 0.975 0.97916667 0.98333333 0.9875 0.99166667 0.99583333 1 1 1 1 1 1